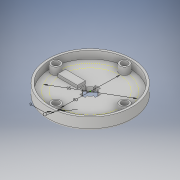
# Autodesk Inventor part: BaseHumedadDireccion
Saved by Autodesk Inventor 2019 (Build 230136000, 136)
## iProperties
Created: 2020-03-30
Part Number: BaseHumedadDireccion
Material: Generic
Document SubType Name: Modeling
Designer: Sergio
Density: 1 g/cm^3
Appearance: Default
Author: Sergio
Autodesk Inventor part; units mm, degrees
ref_plane "YZ Plane" through (0, 0, 0) normal (1, 0, 0) x (0, 1, 0)
ref_plane "XZ Plane" through (0, 0, 0) normal (0, 1, 0) x (-1, 0, 0)
ref_plane "XY Plane" through (0, 0, 0) normal (0, 0, 1) x (1, 0, 0)
sketch "Sketch1" plane through (0, 0, 0) normal (0, 1, 0) x (-1, 0, 0)
  circle A0 centre (0, 0) radius 55
  dimension "d4" = 110
  constraints: 1 centre point
  measures "d4" diameter of A0
sketch "Sketch2" plane through (0, 0, 0) normal (0, 1, 0) x (-1, 0, 0)
  circle A0 centre (0, 0) radius 40 construction
  circle A1 centre (0, 0) radius 47.5 construction
  circle A2 centre (0, 47.5) radius 4.5
  circle A3 centre (0, 47.5) radius 6.5
  dimension "d11" = 95
  dimension "d10" = 80
  dimension "d12" = 9
  dimension "d13" = 13
  constraints: 3 centre point, 3 coincident, 1 vertical alignment, 2 other
  measures "d10" diameter of A0
  measures "d12" diameter of A2
  measures "d13" diameter of A3
extrude "Extrusion1" add sketch "Sketch1" against normal blind 6.6
extrude "Extrusion2" add sketch "Sketch2" along normal blind 10
pattern_circular "Circular Pattern1" count 4 over 360 about axis through (0, -10, 0) along (0, 1, 0) of "Extrusion2"
sketch "Sketch3" plane through (0, -6.6, 0) normal (0, -1, 0) x (1, 0, 0)
  circle A0 centre (0, 0) radius 55
  circle A1 centre (0, 0) radius 55 projected
  circle A2 centre (0, 0) radius 58
  dimension "d21" = 116
  constraints: 2 centre point, 2 coincident, 1 concentric
  measures "d21" diameter of A2
extrude "Extrusion3" add sketch "Sketch3" against normal blind 17
sketch "Sketch4" plane through (0, 0, 0) normal (0, 1, 0) x (1, 0, 0)
  circle A0 centre (0, 0) radius 8.1
  dimension "d24" = 16.2
  constraints: 1 centre point, 1 coincident
  measures "d24" diameter of A0
extrude "Extrusion4" cut sketch "Sketch4" against normal blind 30
sketch "Sketch6" plane through (0, 0, 0) normal (1, 0, 0) x (0, 1, 0)
  line L0 (0, 8.1) -> (0, -8.1) projected
  line L1 (-6.6, -58) -> (-6.6, 58) projected
  line L2 (0, 8.1) -> (-6.6, 8.1)
  line L3 (-6.6, 8.1) -> (-6.6, 11.1)
  line L4 (-6.6, 11.1) -> (0, 11.1)
  line L5 (0, 11.1) -> (0, 8.1)
  line L6 (-8.4, 0) -> (1.4, 0) projected
  point P0 (0, 0)
  dimension "d27" = 3
  constraints: 8 end point, 2 parallel, 1 horizontal, 1 perpendicular, 1 point on line
  measures "d27" distance of L2.end L3.end
revolve "Revolution1" cut sketch "Sketch6" angle 40 mid plane about axis through (0, -10, 0) along (0, 1, 0) contours L2 L1 L4 L5
pattern_circular "Circular Pattern2" count 4 over 360 about axis through (0, -10, 0) along (0, 1, 0) of "Revolution1"
fillet "Fillet1" radius 3 1 edges at (-58, -6.6, 0)
sketch "Sketch7" plane through (0, 0, 0) normal (0, 1, 0) x (1, 0, 0)
  circle A0 centre (0, 0) radius 12.5 construction
  line L0 (-12.144, 5.5) -> (-39.644, 5.5)
  line L1 (-39.644, 5.5) -> (-39.644, -5.5)
  line L2 (-39.644, -5.5) -> (-12.144, -5.5)
  line L3 (-12.144, -5.5) -> (-12.144, 5.5)
  dimension "d33" = 25
  dimension "d34" = 27.5
  dimension "d35" = 11
  dimension "d36" = 5.5
  constraints: 8 end point, 2 parallel, 1 centre point, 1 coincident, 1 horizontal, 1 perpendicular
  measures "d33" diameter of A0
  measures "d34" distance of L2.end L1.end
  measures "d35" distance of L1.end L0.end
  measures "d36" distance from line of point (0, 0) L0
extrude "Extrusion5" add sketch "Sketch7" along normal blind 4
body "Solid1"
